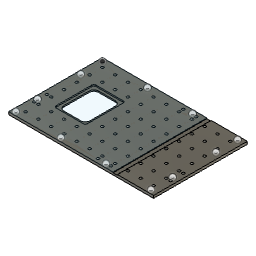
MFT Deluxe Top (Autodesk Fusion 360 design; units mm, degrees)
Autodesk Fusion 360 part; units mm, degrees
sketch "Sketch1" plane through (0, 0, 0) normal (0, 0, 1) x (1, 0, 0)
  line L0 (544, 352) -> (-544, 352)
  line L1 (-544, 352) -> (-544, -352)
  line L2 (-544, -352) -> (544, -352)
  line L3 (544, -352) -> (544, 352)
  circle A0 centre (0, 0) radius 9.95
  circle A1 centre (-576, -384) radius 9.95
  circle A2 centre (-576, -288) radius 9.95
  circle A3 centre (-576, -192) radius 9.95
  circle A4 centre (-576, -96) radius 9.95
  circle A5 centre (-576, 0) radius 9.95
  circle A6 centre (-576, 96) radius 9.95
  circle A7 centre (-576, 192) radius 9.95
  circle A8 centre (-576, 288) radius 9.95
  circle A9 centre (-576, 384) radius 9.95
  circle A10 centre (-480, -384) radius 9.95
  circle A11 centre (-480, -288) radius 9.95
  circle A12 centre (-480, -192) radius 9.95
  circle A13 centre (-480, -96) radius 9.95
  circle A14 centre (-480, 0) radius 9.95
  circle A15 centre (-480, 96) radius 9.95
  circle A16 centre (-480, 192) radius 9.95
  circle A17 centre (-480, 288) radius 9.95
  circle A18 centre (-480, 384) radius 9.95
  circle A19 centre (-384, -384) radius 9.95
  circle A20 centre (-384, -288) radius 9.95
  circle A21 centre (-384, -192) radius 9.95
  circle A22 centre (-384, 192) radius 9.95
  circle A23 centre (-384, 288) radius 9.95
  circle A24 centre (-384, 384) radius 9.95
  circle A25 centre (-288, -384) radius 9.95
  circle A26 centre (-288, -288) radius 9.95
  circle A27 centre (-288, -192) radius 9.95
  circle A28 centre (-288, 192) radius 9.95
  circle A29 centre (-288, 288) radius 9.95
  circle A30 centre (-288, 384) radius 9.95
  circle A31 centre (-192, -384) radius 9.95
  circle A32 centre (-192, -288) radius 9.95
  circle A33 centre (-192, -192) radius 9.95
  circle A34 centre (-192, 192) radius 9.95
  circle A35 centre (-192, 288) radius 9.95
  circle A36 centre (-192, 384) radius 9.95
  circle A37 centre (-96, -384) radius 9.95
  circle A38 centre (-96, -288) radius 9.95
  circle A39 centre (-96, -192) radius 9.95
  circle A40 centre (-96, -96) radius 9.95
  circle A41 centre (-96, 0) radius 9.95
  circle A42 centre (-96, 96) radius 9.95
  circle A43 centre (-96, 192) radius 9.95
  circle A44 centre (-96, 288) radius 9.95
  circle A45 centre (-96, 384) radius 9.95
  circle A46 centre (0, -384) radius 9.95
  circle A47 centre (0, -288) radius 9.95
  circle A48 centre (0, -192) radius 9.95
  circle A49 centre (0, -96) radius 9.95
  circle A50 centre (0, 96) radius 9.95
  circle A51 centre (0, 192) radius 9.95
  circle A52 centre (0, 288) radius 9.95
  circle A53 centre (0, 384) radius 9.95
  circle A54 centre (96, -384) radius 9.95
  circle A55 centre (96, -288) radius 9.95
  circle A56 centre (96, -192) radius 9.95
  circle A57 centre (96, -96) radius 9.95
  circle A58 centre (96, 0) radius 9.95
  circle A59 centre (96, 96) radius 9.95
  circle A60 centre (96, 192) radius 9.95
  circle A61 centre (96, 288) radius 9.95
  circle A62 centre (96, 384) radius 9.95
  circle A63 centre (192, -384) radius 9.95
  circle A64 centre (192, -288) radius 9.95
  circle A65 centre (192, -192) radius 9.95
  circle A66 centre (192, -96) radius 9.95
  circle A67 centre (192, 0) radius 9.95
  circle A68 centre (192, 96) radius 9.95
  circle A69 centre (192, 192) radius 9.95
  circle A70 centre (192, 288) radius 9.95
  circle A71 centre (192, 384) radius 9.95
  circle A72 centre (288, -384) radius 9.95
  circle A73 centre (288, -288) radius 9.95
  circle A74 centre (288, -192) radius 9.95
  circle A75 centre (288, -96) radius 9.95
  circle A76 centre (288, 0) radius 9.95
  circle A77 centre (288, 96) radius 9.95
  circle A78 centre (288, 192) radius 9.95
  circle A79 centre (288, 288) radius 9.95
  circle A80 centre (288, 384) radius 9.95
  circle A81 centre (384, -384) radius 9.95
  circle A82 centre (384, -288) radius 9.95
  circle A83 centre (384, -192) radius 9.95
  circle A84 centre (384, -96) radius 9.95
  circle A85 centre (384, 0) radius 9.95
  circle A86 centre (384, 96) radius 9.95
  circle A87 centre (384, 192) radius 9.95
  circle A88 centre (384, 288) radius 9.95
  circle A89 centre (384, 384) radius 9.95
  circle A90 centre (480, -384) radius 9.95
  circle A91 centre (480, -288) radius 9.95
  circle A92 centre (480, -192) radius 9.95
  circle A93 centre (480, -96) radius 9.95
  circle A94 centre (480, 0) radius 9.95
  circle A95 centre (480, 96) radius 9.95
  circle A96 centre (480, 192) radius 9.95
  circle A97 centre (480, 288) radius 9.95
  circle A98 centre (480, 384) radius 9.95
  circle A99 centre (576, -384) radius 9.95
  circle A100 centre (576, -288) radius 9.95
  circle A101 centre (576, -192) radius 9.95
  circle A102 centre (576, -96) radius 9.95
  circle A103 centre (576, 0) radius 9.95
  circle A104 centre (576, 96) radius 9.95
  circle A105 centre (576, 192) radius 9.95
  circle A106 centre (576, 288) radius 9.95
  circle A107 centre (576, 384) radius 9.95
  circle A108 centre (192, -320) radius 9.95
  circle A109 centre (96, -320) radius 9.95
  circle A110 centre (192, 320) radius 9.95
  circle A111 centre (96, 320) radius 9.95
  circle A112 centre (480, -96) radius 9.95
  circle A113 centre (480, -192) radius 9.95
  circle A114 centre (480, -192) radius 9.95
  circle A115 centre (480, -288) radius 9.95
  circle A116 centre (512, -192) radius 9.95
  circle A117 centre (512, -96) radius 9.95
  circle A118 centre (-512, -192) radius 9.95
  circle A119 centre (-512, -96) radius 9.95
  dimension "d1" = 1088
  dimension "d2" = 704
  dimension "d3" = 19.9
  dimension "d6" = 96
  dimension "d7" = 96
  dimension "d31" = 64
  dimension "d32" = 64
  dimension "d33" = 32
  dimension "d34" = 32
  constraint horizontal L0
  constraint perpendicular L0 L1
  constraint parallel L0 L2
  constraint parallel L1 L3
  constraint coincident A0.centre origin
  measures "d1" distance of L1.end L2.end
  measures "d2" distance of L0.end L1.end
  measures "d3" diameter of A0
  measures "d31" distance of L2 A26.centre
  measures "d32" distance of L1 A14.centre
  measures "d33" distance of L2 A109.centre
  measures "d34" distance of L0 A111.centre
extrude "Extrude1" add sketch "Sketch1" along normal blind 19.05 contours L0 L1 L2 L3 makes body 1
sketch "Sketch2" plane through (0, 0, 19.05) normal (0, 0, 1) x (-1, 0, 0)
  circle A0 centre (-288, 192) radius 9.95
  circle A1 centre (-192, 96) radius 9.95
  circle A2 centre (192, -192) radius 9.95
  circle A3 centre (-480, 288) radius 9.95
  circle A4 centre (-384, -288) radius 9.95
  circle A5 centre (-384, -192) radius 9.95
  circle A6 centre (-384, -96) radius 9.95
  circle A7 centre (-384, 0) radius 9.95
  circle A8 centre (-384, 96) radius 9.95
  circle A9 centre (-192, 0) radius 9.95
  circle A10 centre (-192, -288) radius 9.95
  circle A11 centre (-192, -96) radius 9.95
  circle A12 centre (-192, -192) radius 9.95
  circle A13 centre (-480, 192) radius 9.95
  circle A14 centre (288, 288) radius 9.95
  circle A15 centre (384, -192) radius 9.95
  circle A16 centre (384, -288) radius 9.95
  circle A17 centre (288, 192) radius 9.95
  circle A18 centre (192, 192) radius 9.95
  circle A19 centre (192, 288) radius 9.95
  circle A20 centre (288, -288) radius 9.95
  circle A21 centre (288, -192) radius 9.95
  circle A22 centre (96, 96) radius 9.95
  circle A23 centre (-192, 288) radius 9.95
  circle A24 centre (-480, 0) radius 9.95
  circle A25 centre (96, 0) radius 9.95
  circle A26 centre (-96, 0) radius 9.95
  circle A27 centre (-96, 96) radius 9.95
  circle A28 centre (-192, 192) radius 9.95
  circle A29 centre (-96, -96) radius 9.95
  circle A30 centre (96, 288) radius 9.95
  circle A31 centre (-96, -288) radius 9.95
  circle A32 centre (-96, -192) radius 9.95
  circle A33 centre (192, -288) radius 9.95
  circle A34 centre (96, 192) radius 9.95
  circle A35 centre (0, 96) radius 9.95
  circle A36 centre (0, -288) radius 9.95
  circle A37 centre (0, -192) radius 9.95
  circle A38 centre (-96, 288) radius 9.95
  circle A39 centre (-480, -192) radius 9.95
  circle A40 centre (480, -288) radius 9.95
  circle A41 centre (480, 192) radius 9.95
  circle A42 centre (480, -96) radius 9.95
  circle A43 centre (480, 288) radius 9.95
  circle A44 centre (0, 0) radius 9.95
  circle A45 centre (480, 0) radius 9.95
  circle A46 centre (480, 96) radius 9.95
  circle A47 centre (480, -192) radius 9.95
  circle A48 centre (384, 288) radius 9.95
  circle A49 centre (-384, 288) radius 9.95
  circle A50 centre (0, 288) radius 9.95
  circle A51 centre (384, 192) radius 9.95
  circle A52 centre (0, 192) radius 9.95
  circle A53 centre (0, -96) radius 9.95
  circle A54 centre (96, -96) radius 9.95
  circle A55 centre (96, -192) radius 9.95
  circle A56 centre (-480, 96) radius 9.95
  circle A57 centre (-480, -96) radius 9.95
  circle A58 centre (96, -288) radius 9.95
  circle A59 centre (-480, -288) radius 9.95
  circle A60 centre (-96, 192) radius 9.95
  circle A61 centre (-384, 192) radius 9.95
  circle A62 centre (-288, 96) radius 9.95
  circle A63 centre (-288, -288) radius 9.95
  circle A64 centre (-288, 288) radius 9.95
  circle A65 centre (-288, -192) radius 9.95
  circle A66 centre (-288, -96) radius 9.95
  circle A67 centre (-288, 0) radius 9.95
  line L0 (-544, 352) -> (-544, -352)
  line L1 (-544, -352) -> (544, -352)
  line L2 (544, -352) -> (544, 352)
  line L3 (544, 352) -> (-544, 352)
  line L4 (405.475, 149.225) -> (170.525, 149.225)
  line L5 (170.525, 149.225) -> (170.525, -149.225)
  line L6 (170.525, -149.225) -> (405.475, -149.225)
  line L7 (405.475, -149.225) -> (405.475, 149.225)
  line L8 (405.475, 149.225) -> (170.525, -149.225) construction
  line L9 (170.525, 149.225) -> (405.475, -149.225) construction
  line L10 (386.425, -130.175) -> (386.425, 130.175)
  line L11 (386.425, 130.175) -> (189.575, 130.175)
  line L12 (189.575, 130.175) -> (189.575, -130.175)
  line L13 (189.575, -130.175) -> (386.425, -130.175)
  circle A68 centre (-192, -320) radius 9.95
  circle A69 centre (-96, 320) radius 9.95
  circle A70 centre (-192, 320) radius 9.95
  circle A71 centre (-96, -320) radius 9.95
  circle A72 centre (-512, 192) radius 9.95
  circle A73 centre (-512, 96) radius 9.95
  circle A74 centre (512, 192) radius 9.95
  circle A75 centre (512, 96) radius 9.95
  point P0 (288, 0)
  dimension "d14" = 234.95
  dimension "d15" = 298.45
  dimension "d16" = -19.05
  constraint horizontal L4
  constraint perpendicular L4 L5
  constraint parallel L4 L6
  constraint parallel L5 L7
  constraint coincident L8 P0
  constraint coincident L9 P0
  measures "d14" distance of L5.end L6.end
  measures "d15" distance of L4.end L5.end
extrude "Extrude2" cut sketch "Sketch2" against normal blind 9.525 contours L4 L5 L6 L7 bodies 1
extrude "Extrude3" cut 1 faces at (-320.8083, 43.3917, 19.05) along direction (0, 0, -1) blind 152.4 on bodies 1 bodies 1
fillet "Fillet1" radius 15.875 4 edges at (-405.475, 149.225, 14.2875) (-405.475, -149.225, 14.2875) (-170.525, -149.225, 14.2875) (-170.525, 149.225, 14.2875) on bodies 1
fillet "Fillet3" radius 34.925 4 edges at (-189.575, -130.175, 4.7625) (-189.575, 130.175, 4.7625) (-386.425, 130.175, 4.7625) (-386.425, -130.175, 4.7625) on bodies 1
sketch "Sketch4" plane through (0, 0, 19.05) normal (0, 0, 1) x (-1, 0, 0)
  line L0 (-544, 352) -> (-544, -352)
  line L1 (-544, -352) -> (544, -352)
  line L2 (544, -352) -> (544, 352)
  line L3 (544, 352) -> (-544, 352)
  circle A0 centre (-192, 288) radius 9.95
  circle A1 centre (-192, 192) radius 9.95
  circle A2 centre (-288, -96) radius 9.95
  circle A3 centre (-96, -96) radius 9.95
  circle A4 centre (0, 288) radius 9.95
  circle A5 centre (-96, 96) radius 9.95
  circle A6 centre (-288, 0) radius 9.95
  circle A7 centre (-288, 288) radius 9.95
  circle A8 centre (96, -192) radius 9.95
  circle A9 centre (96, -96) radius 9.95
  circle A10 centre (0, 192) radius 9.95
  circle A11 centre (0, -96) radius 9.95
  circle A12 centre (480, 0) radius 9.95
  circle A13 centre (-288, -192) radius 9.95
  circle A14 centre (-288, 96) radius 9.95
  circle A15 centre (-96, -192) radius 9.95
  circle A16 centre (-96, -288) radius 9.95
  circle A17 centre (0, 96) radius 9.95
  circle A18 centre (-96, 192) radius 9.95
  circle A19 centre (96, 0) radius 9.95
  circle A20 centre (-96, 0) radius 9.95
  circle A21 centre (0, -192) radius 9.95
  circle A22 centre (-288, 192) radius 9.95
  circle A23 centre (0, -288) radius 9.95
  circle A24 centre (96, -288) radius 9.95
  circle A25 centre (-96, 288) radius 9.95
  circle A26 centre (480, -96) radius 9.95
  circle A27 centre (480, 96) radius 9.95
  circle A28 centre (480, -192) radius 9.95
  circle A29 centre (480, 192) radius 9.95
  circle A30 centre (192, -192) radius 9.95
  circle A31 centre (384, 288) radius 9.95
  circle A32 centre (384, 192) radius 9.95
  circle A33 centre (-480, 96) radius 9.95
  circle A34 centre (-480, 0) radius 9.95
  circle A35 centre (-480, -96) radius 9.95
  circle A36 centre (-480, -192) radius 9.95
  circle A37 centre (-480, -288) radius 9.95
  circle A38 centre (96, 192) radius 9.95
  circle A39 centre (192, -288) radius 9.95
  circle A40 centre (96, 288) radius 9.95
  circle A41 centre (96, 96) radius 9.95
  circle A42 centre (-384, 288) radius 9.95
  circle A43 centre (480, 288) radius 9.95
  circle A44 centre (-384, 192) radius 9.95
  circle A45 centre (480, -288) radius 9.95
  circle A46 centre (0, 0) radius 9.95
  circle A47 centre (288, -288) radius 9.95
  circle A48 centre (192, 288) radius 9.95
  circle A49 centre (192, 192) radius 9.95
  circle A50 centre (288, 192) radius 9.95
  circle A51 centre (384, -288) radius 9.95
  circle A52 centre (384, -192) radius 9.95
  circle A53 centre (288, 288) radius 9.95
  circle A54 centre (288, -192) radius 9.95
  circle A55 centre (-192, -192) radius 9.95
  circle A56 centre (-192, -96) radius 9.95
  circle A57 centre (-192, -288) radius 9.95
  circle A58 centre (-384, 96) radius 9.95
  circle A59 centre (-384, 0) radius 9.95
  circle A60 centre (-384, -96) radius 9.95
  circle A61 centre (-384, -192) radius 9.95
  circle A62 centre (-384, -288) radius 9.95
  circle A63 centre (-480, 288) radius 9.95
  circle A64 centre (-480, 192) radius 9.95
  circle A65 centre (-192, 96) radius 9.95
  circle A66 centre (-288, -288) radius 9.95
  circle A67 centre (-192, 0) radius 9.95
  line L4 (186.4, 149.225) -> (389.6, 149.225)
  arc A68 (405.475, 133.35) -> (389.6, 149.225) centre (389.6, 133.35) ccw
  line L5 (405.475, 133.35) -> (405.475, -133.35)
  arc A69 (389.6, -149.225) -> (405.475, -133.35) centre (389.6, -133.35) ccw
  line L6 (389.6, -149.225) -> (186.4, -149.225)
  arc A70 (170.525, -133.35) -> (186.4, -149.225) centre (186.4, -133.35) ccw
  line L7 (170.525, -133.35) -> (170.525, 133.35)
  arc A71 (186.4, 149.225) -> (170.525, 133.35) centre (186.4, 133.35) ccw
  line L8 (-256, -352) -> (-256, 352) construction
  line L9 (-240.125, -352) -> (-271.875, -352)
  line L10 (-271.875, -352) -> (-271.875, 352)
  line L11 (-271.875, 352) -> (-240.125, 352)
  line L12 (-240.125, 352) -> (-240.125, -352)
  circle A72 centre (-96, -320) radius 9.95
  circle A73 centre (-192, 320) radius 9.95
  circle A74 centre (-96, 320) radius 9.95
  circle A75 centre (-192, -320) radius 9.95
  circle A76 centre (512, 96) radius 9.95
  circle A77 centre (512, 192) radius 9.95
  circle A78 centre (-512, 96) radius 9.95
  circle A79 centre (-512, 192) radius 9.95
  dimension "d27" = 64
  dimension "d28" = 31.75
  constraint coincident L1 L8.start
  constraint coincident L3 L8.end
  constraint perpendicular L3 L8
  constraint horizontal L9
  constraint vertical L10
  constraint horizontal L11
  constraint vertical L12
  constraint coincident L1 L9.start
  constraint midpoint L8.start L9
  constraint midpoint L8.end L11
  measures "d27" distance of A57.centre L8
  measures "d28" distance of L9.start L9.end
extrude "Extrude4" cut sketch "Sketch4" against normal blind 4.7625 contours L1 L3 L9 L10 L11 L12 bodies 1
sketch "Sketch5" plane through (0, 0, 19.05) normal (0, 0, 1) x (-1, 0, 0)
  line L0 (-240.125, 352) -> (-240.125, -352)
  line L1 (-240.125, -352) -> (544, -352)
  line L2 (544, -352) -> (544, 352)
  line L3 (544, 352) -> (-240.125, 352)
  circle A0 centre (0, 192) radius 9.95
  circle A1 centre (-96, -320) radius 9.95
  circle A2 centre (512, 96) radius 9.95
  circle A3 centre (-192, -320) radius 9.95
  circle A4 centre (512, 192) radius 9.95
  circle A5 centre (-192, 320) radius 9.95
  circle A6 centre (-96, 320) radius 9.95
  circle A7 centre (96, 0) radius 9.95
  circle A8 centre (96, -96) radius 9.95
  circle A9 centre (96, -192) radius 9.95
  circle A10 centre (96, -288) radius 9.95
  circle A11 centre (-96, -288) radius 9.95
  circle A12 centre (-96, -192) radius 9.95
  circle A13 centre (-96, -96) radius 9.95
  circle A14 centre (-96, 0) radius 9.95
  circle A15 centre (-96, 96) radius 9.95
  circle A16 centre (-96, 192) radius 9.95
  circle A17 centre (-96, 288) radius 9.95
  circle A18 centre (0, -288) radius 9.95
  circle A19 centre (0, -192) radius 9.95
  circle A20 centre (0, -96) radius 9.95
  circle A21 centre (0, 96) radius 9.95
  circle A22 centre (384, -192) radius 9.95
  circle A23 centre (0, 288) radius 9.95
  circle A24 centre (0, 0) radius 9.95
  circle A25 centre (480, 288) radius 9.95
  circle A26 centre (480, 192) radius 9.95
  circle A27 centre (480, 96) radius 9.95
  circle A28 centre (480, 0) radius 9.95
  circle A29 centre (480, -96) radius 9.95
  circle A30 centre (480, -192) radius 9.95
  circle A31 centre (480, -288) radius 9.95
  circle A32 centre (384, 288) radius 9.95
  circle A33 centre (384, 192) radius 9.95
  circle A34 centre (96, 96) radius 9.95
  circle A35 centre (384, -288) radius 9.95
  circle A36 centre (288, 288) radius 9.95
  circle A37 centre (288, 192) radius 9.95
  circle A38 centre (288, -192) radius 9.95
  circle A39 centre (288, -288) radius 9.95
  circle A40 centre (192, 288) radius 9.95
  circle A41 centre (192, 192) radius 9.95
  circle A42 centre (192, -192) radius 9.95
  circle A43 centre (192, -288) radius 9.95
  circle A44 centre (96, 288) radius 9.95
  circle A45 centre (96, 192) radius 9.95
  circle A46 centre (-192, 96) radius 9.95
  circle A47 centre (-192, -192) radius 9.95
  circle A48 centre (-192, -288) radius 9.95
  circle A49 centre (-192, -96) radius 9.95
  circle A50 centre (-192, 288) radius 9.95
  circle A51 centre (-192, 192) radius 9.95
  circle A52 centre (-192, 0) radius 9.95
  line L4 (186.4, 149.225) -> (389.6, 149.225)
  arc A53 (405.475, 133.35) -> (389.6, 149.225) centre (389.6, 133.35) ccw
  line L5 (405.475, 133.35) -> (405.475, -133.35)
  arc A54 (389.6, -149.225) -> (405.475, -133.35) centre (389.6, -133.35) ccw
  line L6 (389.6, -149.225) -> (186.4, -149.225)
  arc A55 (170.525, -133.35) -> (186.4, -149.225) centre (186.4, -133.35) ccw
  line L7 (170.525, -133.35) -> (170.525, 133.35)
  arc A56 (186.4, 149.225) -> (170.525, 133.35) centre (186.4, 133.35) ccw
  point P0 (517, -325)
  point P1 (178.6667, -325)
  point P2 (-159.6667, -325)
  point P3 (-498, -325)
  point P4 (517, -162.5)
  point P5 (-498, -162.5)
  point P6 (517, 162.5)
  point P7 (-498, 162.5)
  point P8 (517, 325)
  point P9 (178.6667, 325)
  point P10 (-159.6667, 325)
  point P11 (-498, 325)
  dimension "d53" = 1015
  dimension "d54" = 650
hole "Hole3" at (-517, 325, 19.05) at (-178.6667, 325, 19.05) at (-517, -325, 19.05) at (-178.6667, -325, 19.05) at (159.6667, -325, 19.05) at (159.6667, 325, 19.05) at (498, 325, 19.05) at (498, -325, 19.05) at (498, -162.5, 19.05) at (498, 162.5, 19.05) at (-517, -162.5, 19.05) at (-517, 162.5, 19.05) direction (0, 0, -1) diameter 6.35 end through all counterbore diameter 19.05 counterbore depth 9.8552 bodies 1
copy_body "Body->Comp1" bodies 1 removing the originals makes body 2 in component "MFT Top"
component "MFT Top" placed x (1, 0, 0) y (0, 1, 0) z (0, 0, 1) at (0, 0, 0)
equation "d8 = ( 3 / 4 ) * 1 in"
equation "d14 = 9 1/4\""
equation "d15 = 11 3/4\""
equation "d17 = ( -3 / 8 ) * 1 in"
equation "d29 = ( -3 / 16 ) * 1 in"
